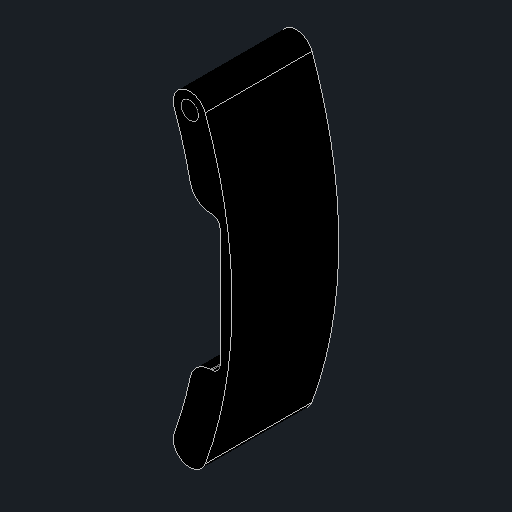
# Autodesk Inventor part: Battery Cover
Saved by Autodesk Inventor 2026.1 (Build 301233020, 233B)
## iProperties
Created: 2026-04-03
Part Number: Battery Cover
Material: Generic
Document SubType Name: Modeling
Designer: Bahaa
Density: 1 g/cm^3
Appearance: Default(1)
Mass: 11.2328 g
Surface Area: 56.3291 cm^2
Volume: 11.2328 cm^3
Author: Bahaa
Autodesk Inventor part; units mm, degrees
ref_plane "YZ Plane" through (0, 0, 0) normal (1, 0, 0) x (0, 1, 0)
ref_plane "XZ Plane" through (0, 0, 0) normal (0, 1, 0) x (-1, 0, 0)
ref_plane "XY Plane" through (0, 0, 0) normal (0, 0, 1) x (1, 0, 0)
derived "Bottom Ring.ipt"
sketch "Sketch5" plane through (0, 0, 0) normal (0, 1, 0) x (1, 0, 0)
  circle A0 centre (0, 0) radius 99.5
  circle A1 centre (0, 0) radius 107.5
  line L0 (95.994, -42.2539) -> (84.1457, -30.4056)
  line L1 (84.1457, 30.4056) -> (95.994, 42.2539)
  circle A2 centre (97.2582, -35.3991) radius 1.6
  circle A3 centre (97.2582, -35.3991) radius 4
  line L2 (99.5, 0) -> (107.5, 0) construction
  line L3 (94.4, -16.35) -> (104.6, -16.35)
  line L4 (104.6, -16.35) -> (104.6, 16.35)
  line L5 (104.6, 16.35) -> (94.4, 16.35)
  line L6 (94.4, 16.35) -> (94.4, -16.35)
  line L7 (94.4, -16.35) -> (104.6, 16.35) construction
  line L8 (104.6, -16.35) -> (94.4, 16.35) construction
  circle A4 centre (97.2582, 35.3991) radius 4
  arc A5 (95.994, 42.2539) -> (96.7662, 46.8247) centre (93.1656, 45.0824) ccw
  arc A6 (96.7662, -46.8247) -> (95.994, -42.2539) centre (93.1656, -45.0824) ccw
  circle A7 centre (97.2582, -35.3991) radius 1.6
  line L9 (88.6408, -34.9007) -> (95.994, -42.2539)
  arc A8 (96.7662, -46.8247) -> (95.994, -42.2539) centre (93.1656, -45.0824) ccw
  arc A9 (96.7662, -46.8247) -> (96.7662, 46.8247) centre (0, 0) ccw
  arc A10 (95.994, 42.2539) -> (96.7662, 46.8247) centre (93.1656, 45.0824) ccw
  line L10 (95.994, 42.2539) -> (88.6408, 34.9007)
  arc A11 (93.5837, 33.7984) -> (88.6408, 34.9007) centre (90.7621, 32.7794) ccw
  arc A12 (97.0576, 21.9106) -> (93.5837, 33.7984) centre (0, 0) ccw
  arc A13 (94.1312, 18.25) -> (97.0576, 21.9106) centre (94.1312, 21.25) ccw
  line L11 (94.1312, 18.25) -> (96.9778, 18.25)
  arc A14 (96.9778, 16.25) -> (96.9778, 18.25) centre (96.9778, 17.25) ccw
  line L12 (96.9778, 16.25) -> (102.5, 16.25)
  arc A15 (104.5, 14.25) -> (102.5, 16.25) centre (102.5, 14.25) ccw
  line L13 (104.5, 14.25) -> (104.5, -14.25)
  arc A16 (102.5, -16.25) -> (104.5, -14.25) centre (102.5, -14.25) ccw
  line L14 (102.5, -16.25) -> (96.9778, -16.25)
  arc A17 (96.9778, -18.25) -> (96.9778, -16.25) centre (96.9778, -17.25) ccw
  line L15 (96.9778, -18.25) -> (94.1312, -18.25)
  arc A18 (97.0576, -21.9106) -> (94.1312, -18.25) centre (94.1312, -21.25) ccw
  arc A19 (93.5837, -33.7984) -> (97.0576, -21.9106) centre (0, 0) ccw
  arc A20 (88.6408, -34.9007) -> (93.5837, -33.7984) centre (90.7621, -32.7794) ccw
  line L16 (91.8941, 38.154) -> (97.9765, 44.2364)
  line L17 (91.8941, -38.154) -> (97.9765, -44.2364)
  point P0 (98.1475, -16.35)
  point P1 (93.4994, -34.031)
  point P2 (101.017, -36.7672)
  point P3 (101.017, 36.7672)
  point P4 (93.4994, 34.031)
  point P5 (98.1475, 16.35)
  constraints: 36 end point, 30 point on circle, 19 centre point, 4 other
extrude "Extrusion1" add sketch "Sketch5" along normal blind 25.8 contours A0 A4 A1 A3 L3 L4 L5 | A4 | A3 | A2
fillet "Fillet1" radius 2 2 edges at (104.6, 12.9, -16.35) (104.6, 12.9, 16.35)
fillet "Fillet2" radius 5 2 edges at (98.1475, 12.9, -16.35) (98.1475, 12.9, 16.35)
sketch "Sketch2" plane through (0, 25.8, 0) normal (0, 1, 0) x (1, 0, 0)
  arc A0 (93.4994, -34.031) -> (101.017, -36.7672) centre (97.2582, -35.3991) ccw projected
  arc A1 (101.017, 36.7672) -> (93.4994, 34.031) centre (97.2582, 35.3991) ccw projected
  point P0 (0, 0)
hole "Hole1" at (97.2582, 25.8, -35.3991) direction (0, -1, 0) diameter 4.2 depth 6
hole "Hole2" at (97.2582, 0, 35.3991) direction (0, 1, 0) diameter 4.2 depth 6
body "Solid1"
